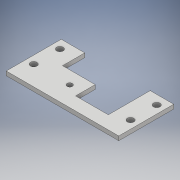
# Autodesk Inventor part: BaseAluminio
Saved by Autodesk Inventor 2018 (Build 220112000, 112)
## iProperties
Created: 2019-05-23
Part Number: BaseAluminio
Material: Generic
Document SubType Name: Modeling
Designer: Ivan
Density: 1 g/cm^3
Appearance: Default
Author: Ivan
Autodesk Inventor part; units mm, degrees
ref_plane "YZ Plane" through (0, 0, 0) normal (1, 0, 0) x (0, 1, 0)
ref_plane "XZ Plane" through (0, 0, 0) normal (0, 1, 0) x (-1, 0, 0)
ref_plane "XY Plane" through (0, 0, 0) normal (0, 0, 1) x (1, 0, 0)
sketch "Sketch1" plane through (0, 0, 0) normal (0, 0, 1) x (1, 0, 0)
  line L0 (-43, 17) -> (43, 17)
  line L1 (43, 17) -> (43, -25)
  line L2 (43, -25) -> (-43, -25)
  line L3 (-43, -25) -> (-43, 17)
  circle A0 centre (-37, 10) radius 2.5
  circle A1 centre (-37, -10) radius 2.5
  line L4 (0, 17) -> (0, -25) construction
  circle A2 centre (37, 10) radius 2.5
  circle A3 centre (37, -10) radius 2.5
  circle A4 centre (-9.5, -10) radius 2
  point P0 (0, 0)
  point P1 (-43, -4)
  dimension "d0" = 86
  dimension "d1" = 42
  dimension "d2" = 5
  dimension "d3" = 7
  dimension "d4" = 6
  dimension "d5" = 6
  dimension "d6" = 15
  dimension "d7" = 4
  dimension "d8" = 27.5
  constraints: 10 end point, 5 centre point, 3 midpoint, 2 parallel, 2 symmetric about line, 1 equal radius, 1 horizontal, 1 horizontal alignment, 1 perpendicular, 1 vertical alignment, 2 other
  measures "d0" distance of L0.start L0.end
  measures "d1" distance of L2.end L0.start
  measures "d2" diameter of A0
  measures "d3" distance from line of L0 A0.centre
  measures "d4" distance from line of L3 A0.centre
  measures "d5" distance from line of L3 A1.centre
  measures "d6" distance from line of L2 A1.centre
  measures "d7" diameter of A4
  measures "d8" distance of A4.centre A1.centre
extrude "Extrusion3" add sketch "Sketch1" along normal blind 3.175
sketch "Sketch3" plane through (0, 0, 3.175) normal (0, 0, 1) x (1, 0, 0)
  line L0 (-25, 17) -> (25, 17)
  line L1 (25, 17) -> (25, 0)
  line L2 (25, 0) -> (-25, 0)
  line L3 (-25, 0) -> (-25, 17)
  line L4 (43, 17) -> (-43, 17) projected
  circle A0 centre (-9.5, -10) radius 2 projected
  line L5 (25, 0) -> (0, 0)
  line L6 (0, 0) -> (0, -15)
  line L7 (0, -15) -> (25, -15)
  line L8 (25, -15) -> (25, 0)
  line L9 (-43, -25) -> (43, -25) projected
  point P0 (0, 0)
  point P1 (0, 17)
  dimension "d20" = 50
  dimension "d22" = 10
  dimension "d23" = 9.5
  dimension "d24" = 10
  constraints: 16 end point, 4 parallel, 2 horizontal, 2 perpendicular, 1 collinear, 1 midpoint, 1 vertical alignment
  measures "d20" distance of L0.start L0.end
  measures "d22" distance from line of L2 A0.centre
  measures "d23" distance from line of A0.centre L6
  measures "d24" distance between parallel lines of L9 L7
extrude "Extrusion4" cut sketch "Sketch3" against normal through all contours L0 L1 L2 L3 | L8 L7 L6 L2
equation "\"d5\" = d4"
equation "\"d24\" = d22"
body "Solid2"
